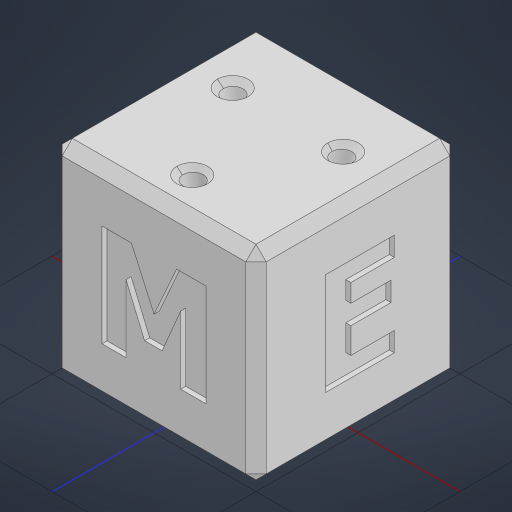
# Autodesk Inventor part: DartCube_Mela
Saved by Autodesk Inventor 2023.2 (Build 272271030, 271C)
## iProperties
Created: 2023-05-18
Part Number: DartCube_Mela
Material: Generisch
Document SubType Name: Modeling
Designer: Stefan
Mass: 61.6566 g
Surface Area: 101.391 cm^2
Volume: 61.6566 cm^3
Density: 1 g/cm^3
Appearance: Vorgabe
Author: Stefan
Autodesk Inventor part; units mm, degrees
ref_plane "YZ Plane" through (0, 0, 0) normal (1, 0, 0) x (0, 1, 0)
ref_plane "XZ Plane" through (0, 0, 0) normal (0, 1, 0) x (-1, 0, 0)
sketch "Skizze1" plane through (0, 0, 0) normal (0, 1, 0) x (-1, 0, 0)
  line L0 (-20, 20) -> (20, 20)
  line L1 (20, 20) -> (20, -20)
  line L2 (20, -20) -> (-20, -20)
  line L3 (-20, -20) -> (-20, 20)
  line L4 (-20, 20) -> (20, -20) construction
  line L5 (20, 20) -> (-20, -20) construction
  point P0 (0, 0)
  dimension "d0" = 40
  constraints: 12 end point, 2 midpoint, 2 parallel, 2 perpendicular, 1 horizontal
  measures "d0" distance of L1.end L2.end
extrude "Extrusion1" add sketch "Skizze1" along normal blind 40
ref_plane "Arbeitsebene2" through (0, 13, 0) normal (0, 1, 0) x (1, 0, 0)
sketch "Skizze8" plane through (0, 40, 0) normal (0, 1, 0) x (1, 0, 0)
  circle A0 centre (0, 0) radius 12.5 construction
  circle A1 centre (0, -12.5) radius 2
  circle A2 centre (10.8253, 6.25) radius 2
  circle A3 centre (-10.8253, 6.25) radius 2
  dimension "d32" = 25
  dimension "d33" = 4
  dimension "d36" = 360
  constraints: 3 centre point, 2 vertical alignment, 1 coincident, 9 other
  measures "d33" diameter of A1
sketch "Skizze9" plane through (0, 13, 0) normal (0, 1, 0) x (1, 0, 0)
  circle A0 centre (0, 0) radius 7.5 construction
  circle A1 centre (0, -7.5) radius 1
  circle A2 centre (6.4952, 3.75) radius 1
  circle A3 centre (-6.4952, 3.75) radius 1
  dimension "d38" = 15
  dimension "d39" = 2
  dimension "d42" = 360
  constraints: 3 centre point, 2 vertical alignment, 1 coincident, 9 other
  measures "d39" diameter of A1
loft "Erhebung1" cut profiles "Skizze8", "Skizze9" contours A1 / A1
loft "Erhebung2" cut profiles "Skizze8", "Skizze9" contours A2 / A2
loft "Erhebung3" cut profiles "Skizze8", "Skizze9" contours A3 / A3
chamfer "Fase1" distance 2 angle 45 12 edges at (20, 20, 20) (20, 40, 0) (0, 40, 20) (0, 40, -20) (20, 20, -20) (0, 0, -20) (20, 0, 0) (-20, 20, -20) (-20, 0, 0) (-20, 40, 0) (-20, 20, 20) (0, 0, 20)
chamfer "Fase2" distance 1 angle 45 3 edges at (-2, 40, 12.5) (-12.8253, 40, -6.25) (8.8253, 40, -6.25)
sketch "Skizze4" plane through (20, 2, 20) normal (0, 0, 1) x (1, 0, 0)
  line L0 (-38, 36) -> (-2, 36) construction
  line L1 (-2, 36) -> (-2, 0) construction
  line L2 (-2, 0) -> (-38, 0) construction
  line L3 (-38, 0) -> (-38, 36) construction
  line L4 (0, 0) -> (0, 0) projected
  line L5 (-38, 36) -> (-2, 36) projected
  line L6 (-2, 36) -> (-2, 0) projected
  line L7 (-2, 0) -> (-38, 0) projected
  line L8 (-38, 0) -> (-38, 36) projected
  line L9 (-9.7893, 8) -> (-14.7812, 8)
  line L10 (-14.7812, 8) -> (-14.7812, 21.2577)
  line L11 (-14.7812, 21.2577) -> (-18.4117, 12.7002)
  line L12 (-18.4117, 12.7002) -> (-21.8477, 12.7002)
  line L13 (-21.8477, 12.7002) -> (-25.4781, 21.2577)
  line L14 (-25.4781, 21.2577) -> (-25.4781, 8)
  line L15 (-25.4781, 8) -> (-30.2107, 8)
  line L16 (-30.2107, 8) -> (-30.2107, 28)
  line L17 (-30.2107, 28) -> (-24.4246, 28)
  line L18 (-24.4246, 28) -> (-19.9838, 18.1297)
  line L19 (-19.9838, 18.1297) -> (-15.5754, 28)
  line L20 (-15.5754, 28) -> (-9.7893, 28)
  line L21 (-9.7893, 28) -> (-9.7893, 8)
  point P0 (-20, -2)
  dimension "d0" = 40
  constraints: 4 collinear, 2 other
sketch "Skizze5" plane through (20, 2, -20) normal (1, 0, 0) x (0, 0, -1)
  line L0 (-38, 36) -> (-2, 36) construction
  line L1 (-2, 36) -> (-2, 0) construction
  line L2 (-2, 0) -> (-38, 0) construction
  line L3 (-38, 0) -> (-38, 36) construction
  line L4 (0, 0) -> (0, 0) projected
  line L5 (-38, 0) -> (-38, 36) projected
  line L6 (-2, 0) -> (-38, 0) projected
  line L7 (-2, 36) -> (-2, 0) projected
  line L8 (-38, 36) -> (-2, 36) projected
  line L9 (-26.3857, 8) -> (-26.3857, 28)
  line L10 (-26.3857, 28) -> (-12.8687, 28)
  line L11 (-12.8687, 28) -> (-12.8687, 24.1912)
  line L12 (-12.8687, 24.1912) -> (-21.3938, 24.1912)
  line L13 (-21.3938, 24.1912) -> (-21.3938, 20.6742)
  line L14 (-21.3938, 20.6742) -> (-13.5332, 20.6742)
  line L15 (-13.5332, 20.6742) -> (-13.5332, 16.8655)
  line L16 (-13.5332, 16.8655) -> (-21.3938, 16.8655)
  line L17 (-21.3938, 16.8655) -> (-21.3938, 11.8088)
  line L18 (-21.3938, 11.8088) -> (-12.8687, 11.8088)
  line L19 (-12.8687, 11.8088) -> (-12.8687, 8)
  line L20 (-12.8687, 8) -> (-26.3857, 8)
  point P0 (-20, -2)
  dimension "d0" = 40
  constraints: 4 collinear, 2 other
sketch "Skizze6" plane through (-20, 2, -20) normal (0, 0, -1) x (-1, 0, 0)
  line L0 (-38, 36) -> (-2, 36) construction
  line L1 (-2, 36) -> (-2, 0) construction
  line L2 (-2, 0) -> (-38, 0) construction
  line L3 (-38, 0) -> (-38, 36) construction
  line L4 (0, 0) -> (0, 0) projected
  line L5 (-38, 36) -> (-2, 36) projected
  line L6 (-38, 0) -> (-38, 36) projected
  line L7 (-2, 0) -> (-38, 0) projected
  line L8 (-2, 36) -> (-2, 0) projected
  line L9 (-12.4554, 8) -> (-25.7942, 8)
  line L10 (-25.7942, 8) -> (-25.7942, 28)
  line L11 (-25.7942, 28) -> (-20.7699, 28)
  line L12 (-20.7699, 28) -> (-20.7699, 11.8088)
  line L13 (-20.7699, 11.8088) -> (-12.4554, 11.8088)
  line L14 (-12.4554, 11.8088) -> (-12.4554, 8)
  point P0 (-20, -2)
  dimension "d0" = 40
  constraints: 4 collinear, 2 other
sketch "Skizze7" plane through (-20, 2, 20) normal (-1, 0, 0) x (0, 0, 1)
  line L0 (-38, 36) -> (-2, 36) construction
  line L1 (-2, 36) -> (-2, 0) construction
  line L2 (-2, 0) -> (-38, 0) construction
  line L3 (-38, 0) -> (-38, 36) construction
  line L4 (0, 0) -> (0, 0) projected
  line L5 (-38, 36) -> (-2, 36) projected
  line L6 (-38, 0) -> (-38, 36) projected
  line L7 (-2, 0) -> (-38, 0) projected
  line L8 (-2, 36) -> (-2, 0) projected
  line L9 (-29.5786, 8) -> (-22.8201, 28)
  line L10 (-22.8201, 28) -> (-17.342, 28)
  line L11 (-17.342, 28) -> (-10.5835, 8)
  line L12 (-10.5835, 8) -> (-15.7536, 8)
  line L13 (-15.7536, 8) -> (-17.0016, 12.0843)
  line L14 (-17.0016, 12.0843) -> (-23.2901, 12.0843)
  line L15 (-23.2901, 12.0843) -> (-24.5543, 8)
  line L16 (-24.5543, 8) -> (-29.5786, 8)
  line L17 (-18.1037, 15.7147) -> (-20.1459, 22.3274)
  line L18 (-20.1459, 22.3274) -> (-22.2042, 15.7147)
  line L19 (-22.2042, 15.7147) -> (-18.1037, 15.7147)
  point P0 (-20, -2)
  dimension "d0" = 40
  constraints: 4 collinear, 2 other
emboss "Prägen1" sketch "Skizze4" operation cut depth 1 direction (0, 0, -1) contours L9 L10 L11 L12 L13 L14 L15 L16 L17 L18 L19 L20 L21
emboss "Prägen2" sketch "Skizze5" operation cut depth 1 direction (-1, 0, 0) contours L9 L10 L11 L12 L13 L14 L15 L16 L17 L18 L19 L20
emboss "Prägen3" sketch "Skizze6" operation cut depth 1 direction (0, 0, 1) contours L9 L10 L11 L12 L13 L14
emboss "Prägen4" sketch "Skizze7" operation cut depth 1 direction (1, 0, 0) contours L9 L10 L11 L12 L13 L14 L15 L16
equation "\"d2\" = d0"
